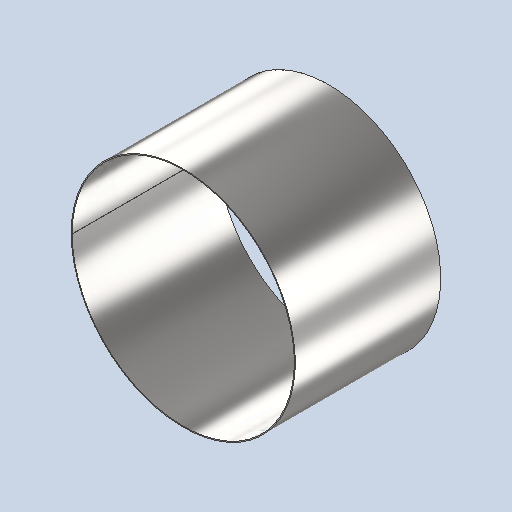
# Autodesk Inventor part: МОО 061 ракета хвост
Saved by Autodesk Inventor 2024.2 (Build 282272000, 272)
## iProperties
Created: 2024-05-19
Part Number: МОО 061 ракета хвост
Material: Stainless Steel
Document SubType Name: Sheet Metal
Designer: admin
Density: 8 g/cm^3
Appearance: Semi-Polished
Flat Pattern Width: 13 cm
Flat Pattern Length: 62.533 cm
Flat Pattern Area: 812.929 cm^2
Sheet Metal Rule: Default
Sheet Metal Width: 130,000 mm
Sheet Metal Length: 625,330 mm
Sheet Metal Area: 81292,889 mm^2
Author: admin
Autodesk Inventor part; units mm, degrees
ref_plane "YZ Plane" through (0, 0, 0) normal (1, 0, 0) x (0, 1, 0)
ref_plane "XZ Plane" through (0, 0, 0) normal (0, 1, 0) x (-1, 0, 0)
ref_plane "XY Plane" through (0, 0, 0) normal (0, 0, 1) x (1, 0, 0)
sketch "Sketch1" plane through (0, 0, 0) normal (0, 0, 1) x (1, 0, 0)
  line L0 (0, 0) -> (0, 130)
  line L1 (-99.2, 130) -> (-100, 130)
  line L2 (-100, 130) -> (-100, 0)
  line L3 (-100, 0) -> (-99.2, 0)
  line L4 (-99.2, 0) -> (-99.2, 130)
  line L5 (-99.2, 130) -> (-100, 0) construction
  line L6 (-100, 130) -> (-99.2, 0) construction
  point P0 (-99.6, 65)
  dimension "d0" = 130
  dimension "d1" = 0.8
  dimension "d2" = 200
  constraints: 14 end point, 2 midpoint, 2 parallel, 2 point on line, 1 horizontal, 1 perpendicular, 1 vertical
  measures "d0" distance of L0.start L0.end
  measures "d1" distance of L1.start L1.end
  measures "d2" diameter of L2 L0
revolve "Revolution1" add sketch "Sketch1" angle 359.9 about axis through (0, 0, 0) along (0, 1, 0)
equation "\"d1\" = Thickness"
equation "\"BendRadius\" = Thickness"
equation "\"BendReliefWidth\" = Thickness"
equation "\"BendReliefDepth\" = 0.5 * Thickness"
equation "\"CornerReliefSize\" = 4 * Thickness"
equation "\"MinimumRemnant\" = 2 * Thickness"
equation "\"TransitionRadius\" = BendRadius"
equation "\"JacobiRadiusSize\" = BendRadius"
equation "\"GapSize\" = Thickness"
equation "\"Thickness\" = 0.8"
body "Solid1"
